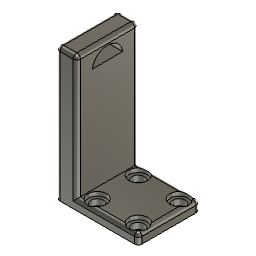
_paper roll mount.a9b0b850-d197-4a2a-a867-633a3fc4cd30 (Autodesk Fusion 360 design; units mm, degrees)
Autodesk Fusion 360 part; units mm, degrees
sketch "Sketch1" plane through (0, 0, 0) normal (0, 0, 1) x (1, 0, 0)
  line L0 (0, 0) -> (40, 0)
  line L1 (40, 0) -> (40, 30)
  line L2 (40, 30) -> (0, 30)
  line L3 (0, 30) -> (0, 0)
  dimension "d1" = 40
  dimension "d2" = 30
  constraint horizontal L0
  constraint vertical L1
  constraint horizontal L2
  constraint vertical L3
  constraint coincident L0.start L3.end
  measures "d1" distance of L0.start L0.end
  measures "d2" distance of L0.start L2.end
extrude "Extrude1" add sketch "Sketch1" along normal blind 5
sketch "Sketch2" plane through (0, 0, 5) normal (0, 0, 1) x (-1, 0, 0)
  line L0 (0, -30) -> (0, 0)
  line L1 (0, 0) -> (-40, 0)
  line L2 (-40, 0) -> (-40, -30)
  line L3 (-40, -30) -> (0, -30)
  line L4 (0, -30) -> (-10, -30)
  line L5 (-10, -30) -> (-10, 0)
  line L6 (-10, 0) -> (0, 0)
  line L7 (0, 0) -> (0, -30)
  dimension "d5" = 10
  dimension "d6" = 30
  constraint horizontal L4
  constraint vertical L5
  constraint horizontal L6
  constraint vertical L7
  constraint coincident L0.start L3.end
  measures "d5" distance of L0.start L4.end
  measures "d6" distance of L0.start L0.end
extrude "Extrude2" add sketch "Sketch2" along normal blind 60 contours L0 L1 L3 L4 L5 L6 L7
sketch "Sketch3" plane through (10, 0, 0) normal (1, 0, 0) x (0, 1, 0)
  line L0 (0, 5) -> (30, 5)
  line L1 (30, 5) -> (30, 65)
  line L2 (30, 65) -> (0, 65)
  line L3 (0, 65) -> (0, 5)
  circle A0 centre (15, 55) radius 7.5
  circle A1 centre (15, 57) radius 7.5
  line L4 (22.5, 55.875) -> (7.5, 55.875)
  line L5 (7.5, 55.875) -> (7.5, 56.125)
  line L6 (7.5, 56.125) -> (22.5, 56.125)
  line L7 (22.5, 56.125) -> (22.5, 55.875)
  line L8 (22.5, 55.875) -> (7.5, 56.125) construction
  line L9 (7.5, 55.875) -> (22.5, 56.125) construction
  point P0 (15, 56)
  dimension "d9" = 15
  dimension "d10" = 15
  dimension "d11" = 15
  dimension "d12" = 0.25
  constraint horizontal L4
  constraint perpendicular L4 L5
  constraint parallel L4 L6
  constraint parallel L5 L7
  constraint coincident L8 P0
  constraint coincident L9 P0
  measures "d9" diameter of A0
  measures "d10" diameter of A1
  measures "d11" distance of L5.end L6.end
  measures "d12" distance of L4.end L5.end
extrude "Extrude3" cut sketch "Sketch3" against normal blind 10 contours A0 L6
sketch "Sketch4" plane through (0, 0, 5) normal (0, 0, 1) x (-1, 0, 0)
  line L0 (-10, -30) -> (-10, 0)
  line L1 (-10, 0) -> (-40, 0)
  line L2 (-40, 0) -> (-40, -30)
  line L3 (-40, -30) -> (-10, -30)
  circle A0 centre (-15, -25) radius 3
  circle A1 centre (-35, -25) radius 3
  circle A2 centre (-15, -5) radius 3
  circle A3 centre (-35, -5) radius 3
  dimension "d17" = 6
  dimension "d18" = 6
  dimension "d19" = 6
  dimension "d20" = 6
  measures "d17" diameter of A0
  measures "d18" diameter of A1
  measures "d19" diameter of A2
  measures "d20" diameter of A3
extrude "Extrude4" cut sketch "Sketch4" against normal blind 5 contours A0 | A1 | A2 | A3
sketch "Sketch5" plane through (0, 0, 5) normal (0, 0, 1) x (-1, 0, 0)
  circle A0 centre (-15, -25) radius 3
  circle A1 centre (-35, -25) radius 3
  circle A2 centre (-15, -5) radius 3
  circle A3 centre (-35, -5) radius 3
  line L0 (-10, -30) -> (-10, 0)
  line L1 (-10, 0) -> (-40, 0)
  line L2 (-40, 0) -> (-40, -30)
  line L3 (-40, -30) -> (-10, -30)
  circle A4 centre (-15, -5) radius 4.5
  circle A5 centre (-15, -25) radius 4.5
  circle A6 centre (-35, -25) radius 4.5
  circle A7 centre (-35, -5) radius 4.5
  dimension "d23" = 9
  dimension "d24" = 9
  dimension "d25" = 9
  dimension "d26" = 9
  constraint concentric A2 A4
  constraint concentric A0 A5
  constraint concentric A1 A6
  constraint concentric A3 A7
  measures "d23" diameter of A4
  measures "d24" diameter of A5
  measures "d25" diameter of A6
  measures "d26" diameter of A7
extrude "Extrude5" cut sketch "Sketch5" against normal blind 2 contours A4 | A5 | A6 | A7
fillet "Fillet1" radius 1.8 13 edges at (5, 0, 65) (0, 15, 65) (10, 15, 65) (10, 0, 35) (0, 0, 32.5) (25, 0, 5) (40, 0, 2.5) (40, 15, 5) (40, 30, 2.5) (25, 30, 5) (10, 30, 35) (0, 30, 32.5) (5, 30, 65)
